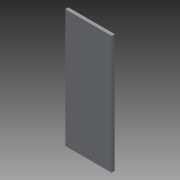
# Autodesk Inventor part: GearPlate
Saved by Autodesk Inventor 2013 (Build 170138000, 138)
## iProperties
Created: 2013-10-25
Part Number: GearPlate
Material: Generic
Document SubType Name: Modeling
Designer: Cody
Density: 1 g/cm^3
Author: Cody
Autodesk Inventor part; units mm, degrees
ref_plane "YZ Plane" through (0, 0, 0) normal (1, 0, 0) x (0, 1, 0)
ref_plane "XZ Plane" through (0, 0, 0) normal (0, 1, 0) x (-1, 0, 0)
ref_plane "XY Plane" through (0, 0, 0) normal (0, 0, 1) x (1, 0, 0)
sketch "Sketch1" plane through (0, 0, 0) normal (0, 0, 1) x (1, 0, 0)
  line L0 (-19.05, -36.0045) -> (19.05, -36.0045)
  line L1 (19.05, -36.0045) -> (19.05, 36.0045)
  line L2 (19.05, 36.0045) -> (-19.05, 36.0045)
  line L3 (-19.05, 36.0045) -> (-19.05, -36.0045)
  line L4 (-19.05, -36.0045) -> (19.05, 36.0045) construction
  line L5 (19.05, -36.0045) -> (-19.05, 36.0045) construction
  point P0 (0, 0)
  dimension "d0" = 38.1
  dimension "d1" = 72.009
  constraints: 12 end point, 2 midpoint, 2 parallel, 1 horizontal, 1 perpendicular
  measures "d0" distance of L2.end L1.end
  measures "d1" distance of L1.end L0.end
extrude "Extrusion1" add sketch "Sketch1" along normal blind 2.54
sketch "Sketch2" plane through (0, 0, 2.54) normal (0, 0, 1) x (1, 0, 0)
  circle A0 centre (-12.7, 23.3045) radius 1.85 projected
  circle A1 centre (12.7, 23.3045) radius 1.85 projected
  circle A2 centre (-12.7, -23.3045) radius 1.85 projected
  circle A3 centre (12.7, -23.3045) radius 1.85 projected
  point P0 (0, 0)
extrude "Extrusion2" cut sketch "Sketch2" against normal blind 2.54
body "Solid1"
